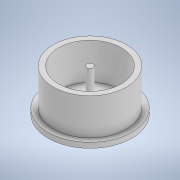
# Autodesk Inventor part: new base
Saved by Autodesk Inventor 2022 (Build 260153000, 153)
## iProperties
Created: 2022-01-28
Part Number: new base
Material: Generic
Document SubType Name: Modeling
Designer: Alexa
Density: 1 g/cm^3
Appearance: Default
Author: Alexa
Autodesk Inventor part; units mm, degrees
ref_plane "YZ Plane" through (0, 0, 0) normal (1, 0, 0) x (0, 1, 0)
ref_plane "XZ Plane" through (0, 0, 0) normal (0, 1, 0) x (-1, 0, 0)
ref_plane "XY Plane" through (0, 0, 0) normal (0, 0, 1) x (1, 0, 0)
sketch "Sketch1" plane through (0, 0, 0) normal (0, 1, 0) x (-1, 0, 0)
  circle A0 centre (0, 0) radius 80
  dimension "d0" = 160
  constraints: 1 centre point, 1 coincident
  measures "d0" diameter of A0
extrude "Extrusion1" add sketch "Sketch1" along normal blind 10
sketch "Sketch2" plane through (0, 10, 0) normal (0, 1, 0) x (1, 0, 0)
  circle A0 centre (0, 0) radius 70
  circle A1 centre (0, 0) radius 60
  circle A2 centre (0, 0) radius 6
  dimension "d3" = 140
  dimension "d4" = 120
  dimension "d5" = 12
  constraints: 3 centre point, 3 coincident
  measures "d3" diameter of A0
  measures "d4" diameter of A1
  measures "d5" diameter of A2
extrude "Extrusion2" add sketch "Sketch2" along normal blind 70
body "Solid1"
